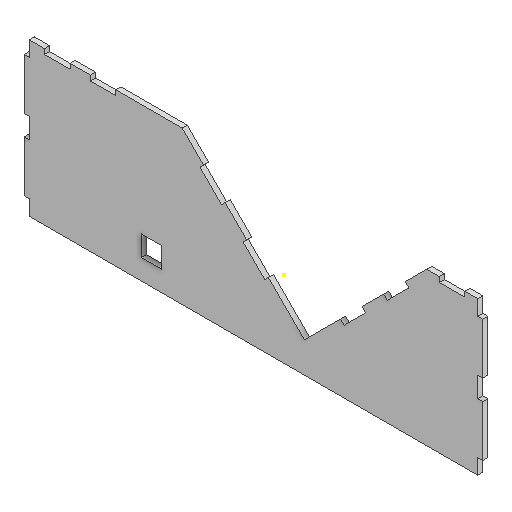
# Autodesk Inventor part: Fondo
Saved by Autodesk Inventor 2022 (Build 260153000, 153)
## iProperties
Created: 2022-06-06
Part Number: Fondo
Material: Generic
Document SubType Name: Modeling
Designer: ADMIN
Density: 1 g/cm^3
Appearance: Default
Author: ADMIN
Autodesk Inventor part; units mm, degrees
ref_plane "YZ Plane" through (0, 0, 0) normal (1, 0, 0) x (0, 1, 0)
ref_plane "XZ Plane" through (0, 0, 0) normal (0, 1, 0) x (-1, 0, 0)
ref_plane "XY Plane" through (0, 0, 0) normal (0, 0, 1) x (1, 0, 0)
sketch "Sketch1" plane through (0, 0, 0) normal (0, 0, 1) x (1, 0, 0)
  line L0 (190, -75) -> (-250, -75) projected
  line L1 (190, 75) -> (190, -75) projected
  line L2 (-250, 75) -> (-235, 75) projected
  line L3 (-250, -75) -> (-250, 75) projected
  line L4 (-255, -10) -> (-255, -60) projected
  line L5 (-255, -60) -> (-250, -60) projected
  line L6 (-250, -10) -> (-250, -60) projected
  line L7 (-255, -10) -> (-250, -10) projected
  line L8 (-255, 60) -> (-255, 10) projected
  line L9 (-255, 10) -> (-250, 10) projected
  line L10 (-250, 60) -> (-250, 10) projected
  line L11 (-255, 60) -> (-250, 60) projected
  line L12 (190, 60) -> (190, 10) projected
  line L13 (190, 10) -> (195, 10) projected
  line L14 (195, 60) -> (195, 10) projected
  line L15 (190, 60) -> (195, 60) projected
  line L16 (190, -10) -> (190, -60) projected
  line L17 (190, -60) -> (195, -60) projected
  line L18 (195, -10) -> (195, -60) projected
  line L19 (190, -10) -> (195, -10) projected
  line L20 (140, 75) -> (152.5, 75) projected
  line L21 (20, -45) -> (55.3553, -9.6447) projected
  line L22 (-100, 75) -> (-78.9949, 53.9949) projected
  line L23 (-15.3553, -9.6447) -> (-18.8909, -13.1802) projected
  line L24 (-18.8909, -13.1802) -> (-40.1041, 8.033) projected
  line L25 (-40.1041, 8.033) -> (-36.5685, 11.5685) projected
  line L26 (-57.7817, 32.7817) -> (-36.5685, 11.5685) projected
  line L27 (-57.7817, 32.7817) -> (-61.3173, 29.2462) projected
  line L28 (-61.3173, 29.2462) -> (-82.5305, 50.4594) projected
  line L29 (-82.5305, 50.4594) -> (-78.9949, 53.9949) projected
  line L30 (118.9949, 53.9949) -> (140, 75) projected
  line L31 (118.9949, 53.9949) -> (122.5305, 50.4594) projected
  line L32 (122.5305, 50.4594) -> (101.3173, 29.2462) projected
  line L33 (101.3173, 29.2462) -> (97.7817, 32.7817) projected
  line L34 (76.5685, 11.5685) -> (97.7817, 32.7817) projected
  line L35 (76.5685, 11.5685) -> (80.1041, 8.033) projected
  line L36 (80.1041, 8.033) -> (58.8909, -13.1802) projected
  line L37 (58.8909, -13.1802) -> (55.3553, -9.6447) projected
  line L38 (-15.3553, -9.6447) -> (20, -45) projected
  line L39 (-210, 75) -> (-210, 70) projected
  line L40 (-210, 70) -> (-235, 70) projected
  line L41 (-235, 70) -> (-235, 75) projected
  line L42 (177.5, 75) -> (190, 75) projected
  line L43 (177.5, 75) -> (177.5, 70) projected
  line L44 (177.5, 70) -> (152.5, 70) projected
  line L45 (152.5, 70) -> (152.5, 75) projected
  line L46 (-165, 75) -> (-100, 75) projected
  line L47 (-165, 75) -> (-165, 70) projected
  line L48 (-165, 70) -> (-190, 70) projected
  line L49 (-190, 70) -> (-190, 75) projected
  line L50 (-210, 75) -> (-190, 75) projected
  point P0 (0, 0)
extrude "Extrusion1" add sketch "Sketch1" along normal blind 5
sketch "Sketch2" plane through (0, 0, 5) normal (0, 0, 1) x (1, 0, 0)
  point P0 (0, 0)
sketch "Sketch4" plane through (0, 0, 5) normal (0, 0, 1) x (1, 0, 0)
  line L0 (190, -60) -> (195, -60) projected
  line L1 (195, -60) -> (195, -10) projected
  line L2 (195, -10) -> (190, -10) projected
  line L3 (190, -10) -> (190, 10) projected
  line L4 (190, 10) -> (195, 10) projected
  line L5 (195, 10) -> (195, 60) projected
  line L6 (195, 60) -> (190, 60) projected
  line L7 (190, 60) -> (190, 75) projected
  line L8 (190, 75) -> (177.5, 75) projected
  line L9 (177.5, 75) -> (177.5, 70) projected
  line L10 (177.5, 70) -> (152.5, 70) projected
  line L11 (152.5, 70) -> (152.5, 75) projected
  line L12 (152.5, 75) -> (140, 75) projected
  line L13 (140, 75) -> (118.9949, 53.9949) projected
  line L14 (118.9949, 53.9949) -> (122.5305, 50.4594) projected
  line L15 (122.5305, 50.4594) -> (101.3173, 29.2462) projected
  line L16 (101.3173, 29.2462) -> (97.7817, 32.7817) projected
  line L17 (97.7817, 32.7817) -> (76.5685, 11.5685) projected
  line L18 (76.5685, 11.5685) -> (80.1041, 8.033) projected
  line L19 (80.1041, 8.033) -> (58.8909, -13.1802) projected
  line L20 (58.8909, -13.1802) -> (55.3553, -9.6447) projected
  line L21 (55.3553, -9.6447) -> (20, -45) projected
  line L22 (20, -45) -> (-15.3553, -9.6447) projected
  line L23 (-15.3553, -9.6447) -> (-18.8909, -13.1802) projected
  line L24 (-18.8909, -13.1802) -> (-40.1041, 8.033) projected
  line L25 (-40.1041, 8.033) -> (-36.5685, 11.5685) projected
  line L26 (-36.5685, 11.5685) -> (-57.7817, 32.7817) projected
  line L27 (-57.7817, 32.7817) -> (-61.3173, 29.2462) projected
  line L28 (-61.3173, 29.2462) -> (-82.5305, 50.4594) projected
  line L29 (-82.5305, 50.4594) -> (-78.9949, 53.9949) projected
  line L30 (-78.9949, 53.9949) -> (-100, 75) projected
  line L31 (-100, 75) -> (-165, 75) projected
  line L32 (-165, 75) -> (-165, 70) projected
  line L33 (-165, 70) -> (-190, 70) projected
  line L34 (-190, 70) -> (-190, 75) projected
  line L35 (-190, 75) -> (-210, 75) projected
  line L36 (-210, 75) -> (-210, 70) projected
  line L37 (-210, 70) -> (-235, 70) projected
  line L38 (-235, 70) -> (-235, 75) projected
  line L39 (-235, 75) -> (-250, 75) projected
  line L40 (-250, 75) -> (-250, 60) projected
  line L41 (-250, 60) -> (-255, 60) projected
  line L42 (-255, 60) -> (-255, 10) projected
  line L43 (-255, 10) -> (-250, 10) projected
  line L44 (-250, 10) -> (-250, -10) projected
  line L45 (-250, -10) -> (-255, -10) projected
  line L46 (-255, -10) -> (-255, -60) projected
  line L47 (-255, -60) -> (-250, -60) projected
  line L48 (-250, -60) -> (-250, -75) projected
  line L49 (-250, -75) -> (190, -75) projected
  line L50 (190, -75) -> (190, -60) projected
  line L51 (-140, -35) -> (-120, -35)
  line L52 (-120, -35) -> (-120, -55)
  line L53 (-120, -55) -> (-140, -55)
  line L54 (-140, -55) -> (-140, -35)
  point P0 (0, 0)
  dimension "d4" = 20
  dimension "d5" = 20
  dimension "d6" = 20
  dimension "d7" = 110
  constraints: 8 end point, 2 parallel, 1 horizontal, 1 perpendicular
  measures "d4" distance of L52.end L53.end
  measures "d5" distance of L51.end L52.end
  measures "d6" distance between parallel lines of L49 L53
  measures "d7" distance between parallel lines of L48 L54
extrude "Extrusion3" cut sketch "Sketch4" against normal blind 10 contours L51 L52 L53 L54
body "Solid1"
